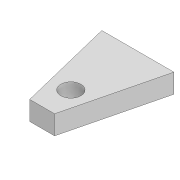
# Autodesk Inventor part: Clamp
Saved by Autodesk Inventor 2020 (Build 240168000, 168)
## iProperties
Created: 2022-03-01
Part Number: Clamp
Material: Generic
Document SubType Name: Modeling
Designer: ferrerx
Density: 1 g/cm^3
Appearance: Default
Author: ferrerx
Autodesk Inventor part; units mm, degrees
ref_plane "YZ Plane" through (0, 0, 0) normal (1, 0, 0) x (0, 1, 0)
ref_plane "XZ Plane" through (0, 0, 0) normal (0, 1, 0) x (-1, 0, 0)
ref_plane "XY Plane" through (0, 0, 0) normal (0, 0, 1) x (1, 0, 0)
sketch "Sketch1" plane through (0, 0, 0) normal (0, 1, 0) x (-1, 0, 0)
  circle A0 centre (0, 0) radius 1.05
  line L0 (5, 20) -> (-5, 20)
  line L1 (-5, 20) -> (-5, -5)
  line L2 (-5, -5) -> (5, -5)
  line L3 (5, -5) -> (5, 20)
  circle A1 centre (0, 15) radius 1.05
  dimension "d0" = 2.1
  dimension "d1" = 5
  dimension "d2" = 10
  dimension "d4" = 5
  dimension "d16" = 2.1
  dimension "d17" = 15
  dimension "d18" = 5
  constraints: 8 end point, 2 centre point, 2 parallel, 1 coincident, 1 horizontal, 1 perpendicular
  measures "d0" diameter of A0
  measures "d1" distance from line of L1 A0.centre
  measures "d2" distance of L1.end L2.end
  measures "d4" distance from line of L2 A0.centre
  measures "d16" diameter of A1
  measures "d17" distance of A0.centre A1.centre
  measures "d18" distance from line of L0 A1.centre
extrude "Extrusion1" add sketch "Sketch1" along normal blind 10
sketch "Sketch2" plane through (5, 0, 20) normal (1, 0, 0) x (0, 0, -1)
  line L0 (0, 10) -> (25, 10) projected
  line L1 (15, 10) -> (17.5478, 3)
  line L2 (17.5478, 3) -> (25, 3)
  line L3 (18.95, 10) -> (18.95, 0) projected
  line L4 (25, 3) -> (25, 10)
  line L5 (25, 10) -> (15, 10)
  line L6 (25, 0) -> (25, 10) projected
  line L7 (0, 0) -> (25, 0) projected
  point P0 (20, 0)
  dimension "d8" = 3
  dimension "d9" = 110
  dimension "d10" = 10
  constraints: 8 end point, 3 perpendicular, 1 collinear, 1 point on line
  measures "d8" distance between parallel lines of L7 L2
  measures "d9" angle of L2 L1
  measures "d10" distance of L0.end L1.start
extrude "Extrusion2" cut sketch "Sketch2" against normal blind 10 contours L0 L3 L2 L1 | L0 L4 L2 L3
sketch "Sketch3" plane through (0, 10, 0) normal (0, 1, 0) x (1, 0, 0)
  circle A0 centre (0, 0) radius 2
  dimension "d13" = 4
  constraints: 1 centre point, 1 coincident
  measures "d13" diameter of A0
extrude "Extrusion3" cut sketch "Sketch3" against normal up to surface (7 mm away)
sketch "Sketch4" plane through (0, 10, 0) normal (0, 1, 0) x (1, 0, 0)
  circle A0 centre (0, -15) radius 1.05 projected
  circle A1 centre (0, -15) radius 2.25
  point P0 (0, 0)
  dimension "d19" = 4.5
  constraints: 1 centre point, 1 coincident
  measures "d19" diameter of A1
extrude "Extrusion4" cut sketch "Sketch4" against normal up to surface (7 mm away)
chamfer "Chamfer1" distance 1 angle 45 1 edges at (1.05, 3, 0)
sketch "Sketch5" plane through (5, 0, -5) normal (0, 0, -1) x (-1, 0, 0)
  line L0 (5, 0) -> (5, 5.666) construction
  circle A0 centre (5, 5.666) radius 2.1
  line L1 (10, 3) -> (0, 3) projected
  dimension "d25" = 4.2
  dimension "d26" = 2.666
  constraints: 2 end point, 1 centre point, 1 coincident, 1 vertical
  measures "d25" diameter of A0
  measures "d26" distance from line of L1 A0.centre
extrude "Extrusion5" cut sketch "Sketch5" against normal blind 31.5
sketch "Sketch6" plane through (0, 10, 0) normal (0, 1, 0) x (1, 0, 0)
  line L0 (5, -5) -> (-5, -5) projected
  line L1 (0, -5) -> (0, -20) construction
  line L2 (-5, -20) -> (5, -20) projected
  line L3 (3.45, -10.575) -> (-3.45, -10.575)
  line L4 (-3.45, -10.575) -> (-3.45, -7.425)
  line L5 (-3.45, -7.425) -> (3.45, -7.425)
  line L6 (3.45, -7.425) -> (3.45, -10.575)
  line L7 (3.45, -10.575) -> (-3.45, -7.425) construction
  line L8 (-3.45, -10.575) -> (3.45, -7.425) construction
  point P0 (0, 0)
  point P1 (0, -9)
  dimension "d29" = 6.9
  dimension "d30" = 3.15
  dimension "d31" = 4
  constraints: 14 end point, 4 midpoint, 2 parallel, 1 horizontal, 1 perpendicular, 1 point on line, 1 vertical
  measures "d29" distance of L4.end L5.end
  measures "d30" distance of L3.end L4.end
  measures "d31" distance from line of L0 point (0, -9)
extrude "Extrusion6" cut sketch "Sketch6" against normal blind 5
sketch "Sketch7" plane through (-3.45, 10, 7.425) normal (0, 0, 1) x (1, 0, 0)
  arc A0 (5.4416, -5) -> (1.4584, -5) centre (3.45, -4.334) ccw projected
  line L0 (3.45, -8.3177) -> (0, -6.3259)
  line L1 (0, -6.3259) -> (0, -2.3421)
  line L2 (0, -2.3421) -> (3.45, -0.3503)
  line L3 (3.45, -0.3503) -> (6.9, -2.3421)
  line L4 (6.9, -2.3421) -> (6.9, -6.3259)
  line L5 (6.9, -6.3259) -> (3.45, -8.3177)
  point P0 (3.45, -10)
  dimension "d34" = 6.9
  constraints: 12 end point, 1 coincident, 13 other
  measures "d34" distance between parallel lines of L4 L1
extrude "Extrusion7" cut sketch "Sketch7" along normal blind 3.15
sketch "Sketch8" plane through (-5, 0, 20) normal (0, 0, 1) x (1, 0, 0)
  line L0 (0, 10) -> (10, 10)
  line L1 (10, 10) -> (10, 8)
  line L2 (10, 8) -> (0, 8)
  line L3 (0, 8) -> (0, 10)
  line L4 (0, 10) -> (10, 10) projected
  line L5 (10, 0) -> (10, 10) projected
  line L6 (0, 0) -> (0, 10) projected
  point P0 (5, 0)
  dimension "d37" = 2
  constraints: 8 end point, 3 collinear, 2 parallel, 1 horizontal, 1 perpendicular
  measures "d37" distance of L0.end L1.end
extrude "Extrusion8" add sketch "Sketch8" along normal blind 28
chamfer "Chamfer2" distance 4 angle 45 1 edges at (0, 8, 20)
sketch "Sketch9" plane through (0, 10, 0) normal (0, 1, 0) x (1, 0, 0)
  circle A0 centre (0, -45) radius 1.05
  line L0 (5, -48) -> (-5, -48) projected
  point P0 (0, 0)
  dimension "d46" = 2.1
  dimension "d50" = 3
  constraints: 1 centre point
  measures "d46" diameter of A0
  measures "d50" distance from line of L0 A0.centre
extrude "Extrusion9" cut sketch "Sketch9" against normal blind 15
sketch "Sketch10" plane through (0, 10, 0) normal (0, 1, 0) x (1, 0, 0)
  line L0 (5, -48) -> (-5, -48) projected
  line L1 (-1.3, -48) -> (-5, -33)
  line L2 (-5, -5) -> (-5, -48) projected
  line L3 (-5, -33) -> (-5, -48)
  line L4 (-5, -48) -> (-1.3, -48)
  line L5 (0, -35) -> (0, 5) construction
  line L6 (1.3, -48) -> (5, -33)
  line L7 (5, -33) -> (5, -48)
  line L8 (5, -48) -> (1.3, -48)
  point P0 (0, 0)
  dimension "d51" = 1.3
  dimension "d52" = 15
  constraints: 14 end point, 2 point on line, 2 symmetric about line, 1 perpendicular
  measures "d51" distance from line of L5 L1.start
  measures "d52" distance from line of L1.end L0
extrude "Extrusion10" cut sketch "Sketch10" against normal blind 15
sketch "Sketch11" plane through (0, 10, 0) normal (0, 1, 0) x (1, 0, 0)
  line L0 (-5, 5) -> (-5, -20) projected
  line L1 (-5, 5) -> (5, 5)
  line L2 (5, 5) -> (5, -38)
  line L3 (5, -38) -> (-5, -38)
  line L4 (-5, -38) -> (-5, 5)
  line L5 (1.3, -48) -> (-1.3, -48) projected
  line L6 (5, -5) -> (5, -33) projected
  point P0 (0, 0)
  dimension "d55" = 10
  constraints: 8 end point, 2 parallel, 1 collinear, 1 horizontal, 1 perpendicular
  measures "d55" distance between parallel lines of L5 L3
extrude "Extrusion11" cut sketch "Sketch11" against normal blind 10
body "Solid1"
